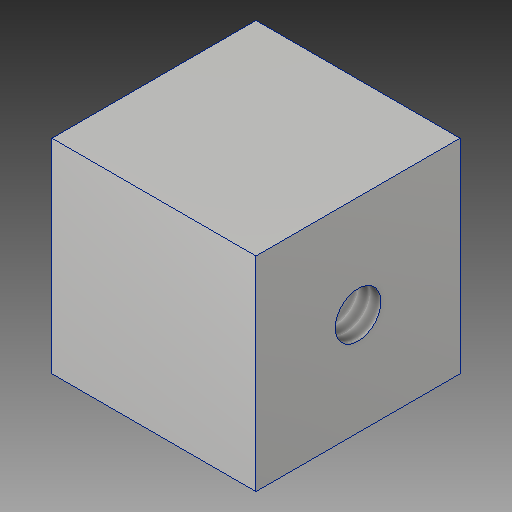
# Autodesk Inventor part: FRA_009_SideCenterPlug
Saved by Autodesk Inventor 2018 (Build 220112000, 112)
## iProperties
Created: 2020-01-22
Part Number: FRA_009_SideCenterPlug
Material: Aluminum 6061
Document SubType Name: Modeling
Designer: 22turnmaxw
Density: 2.7 g/cm^3
Appearance: Aluminum - Flat
Mass: 28.4727 g
Surface Area: 32.7237 cm^2
Volume: 10.5454 cm^3
Author: 22turnmaxw
Autodesk Inventor part; units mm, degrees
ref_plane "YZ Plane" through (0, 0, 0) normal (1, 0, 0) x (0, 1, 0)
ref_plane "XZ Plane" through (0, 0, 0) normal (0, 1, 0) x (-1, 0, 0)
ref_plane "XY Plane" through (0, 0, 0) normal (0, 0, 1) x (1, 0, 0)
sketch "Sketch1" plane through (0, 0, 0) normal (0, 0, 1) x (1, 0, 0)
  line L0 (0, 0) -> (22.225, 0)
  line L1 (22.225, 0) -> (22.225, 22.225)
  line L2 (22.225, 22.225) -> (0, 22.225)
  line L3 (0, 22.225) -> (0, 0)
  dimension "d0" = 22.225
  constraints: 8 end point, 2 parallel, 2 perpendicular, 1 horizontal
  measures "d0" distance of L1.end L2.end
extrude "Extrusion1" add sketch "Sketch1" along normal blind 22.225
sketch "Sketch2" plane through (22.225, 0, 0) normal (1, 0, 0) x (0, 0, -1)
  line L0 (0, 22.225) -> (-22.225, 22.225) projected
  line L1 (0, 0) -> (0, 22.225) projected
  point P0 (-11.1125, 11.1125)
  dimension "d3" = 11.1125
  dimension "d4" = 11.1125
  measures "d3" distance from line of L0 point (-11.113, 11.113)
  measures "d4" distance from line of L1 point (-11.113, 11.113)
hole "Hole1" at (22.225, 11.1125, 11.1125) direction (-1, 0, 0) diameter 4.9784 end through all thread size "1/4-20 UNC" class "2B" standard "ANSI Unified Screw Threads"
body "Solid1"
